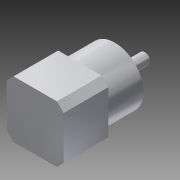
# Autodesk Inventor part: StepperMotorNema17Geared
Saved by Autodesk Inventor 2015 (Build 190159000, 159)
## iProperties
Created: 2014-08-16
Part Number: StepperMotorNema17Geared
Material: Aluminum 6061
Document SubType Name: Modeling
Designer: Jack
Density: 2.7 g/cm^3
Appearance: Aluminum - Flat
Author: Jack
Autodesk Inventor part; units mm, degrees
ref_plane "YZ Plane" through (0, 0, 0) normal (1, 0, 0) x (0, 1, 0)
ref_plane "XZ Plane" through (0, 0, 0) normal (0, 1, 0) x (-1, 0, 0)
ref_plane "XY Plane" through (0, 0, 0) normal (0, 0, 1) x (1, 0, 0)
sketch "Sketch1" plane through (0, 0, 0) normal (0, 1, 0) x (-1, 0, 0)
  line L0 (0, 0) -> (0, -42)
  line L1 (0, -42) -> (42, -42)
  line L2 (42, -42) -> (42, 0)
  line L3 (42, 0) -> (0, 0)
  dimension "d0" = 42
  dimension "d1" = 42
  constraints: 8 end point, 2 parallel, 1 perpendicular, 1 vertical
  measures "d0" distance of L0.start L0.end
  measures "d1" distance of L1.end L0.end
extrude "Extrusion1" add sketch "Sketch1" along normal blind 33
chamfer "Chamfer1" distance 5 angle 45 4 edges at (0, 16.5, 0) (-42, 16.5, 0) (-42, 16.5, -42) (0, 16.5, -42)
sketch "Sketch2" plane through (0, 33, 0) normal (0, 1, 0) x (1, 0, 0)
  line L0 (-5, 42) -> (-37, 42) projected
  line L1 (0, 5) -> (0, 37) projected
  circle A0 centre (-21, 21) radius 21
  point P0 (0, 0)
  dimension "d4" = 5
  dimension "d7" = 42
  dimension "d8" = 21
  dimension "d9" = 21
  constraints: 1 centre point
  measures "d7" diameter of A0
  measures "d8" distance from line of L0 A0.centre
  measures "d9" distance from line of L1 A0.centre
extrude "Extrusion2" add sketch "Sketch2" along normal blind 26
sketch "Sketch3" plane through (-21, 59, -21) normal (0, 1, 0) x (1, 0, 0)
  circle A0 centre (0, 0) radius 21 projected
  line L0 (11.5, 4.899) -> (11.5, -4.899)
  line L1 (-11.5, 4.899) -> (-11.5, -4.899)
  arc A1 (-11.5, -4.899) -> (11.5, -4.899) centre (0, 0) ccw
  arc A2 (11.5, 4.899) -> (-11.5, 4.899) centre (0, 0) ccw
  point P0 (21, -21)
  dimension "d13" = 11.5
  dimension "d14" = 11.5
  dimension "d15" = 12.5
  dimension "d16" = 12.5
  constraints: 4 end point, 4 point on circle, 2 centre point, 1 coincident, 1 parallel, 1 vertical
  measures "d13" distance from line of A0.centre L1
  measures "d14" distance from line of A0.centre L0
  measures "d15" radius of A2
  measures "d16" radius of A1
extrude "Extrusion3" add sketch "Sketch3" along normal blind 2 contours L0 A1 L1 A2
sketch "Sketch4" plane through (-21, 61, -21) normal (0, 1, 0) x (1, 0, 0)
  arc A0 (11.5, 4.899) -> (-11.5, 4.899) centre (0, 0) ccw projected
  arc A1 (-11.5, -4.899) -> (11.5, -4.899) centre (0, 0) ccw projected
  arc A2 (3.5, 1.9365) -> (3.5, -1.9365) centre (0, 0) ccw
  line L0 (3.5, 1.9365) -> (3.5, -1.9365)
  point P0 (21, -21)
  dimension "d19" = 8
  dimension "d20" = 3.5
  constraints: 2 end point, 2 point on circle, 1 centre point, 1 coincident, 1 vertical
  measures "d19" diameter of A2
  measures "d20" distance from line of A0.centre L0
extrude "Extrusion4" add sketch "Sketch4" along normal blind 20
body "Solid1"
